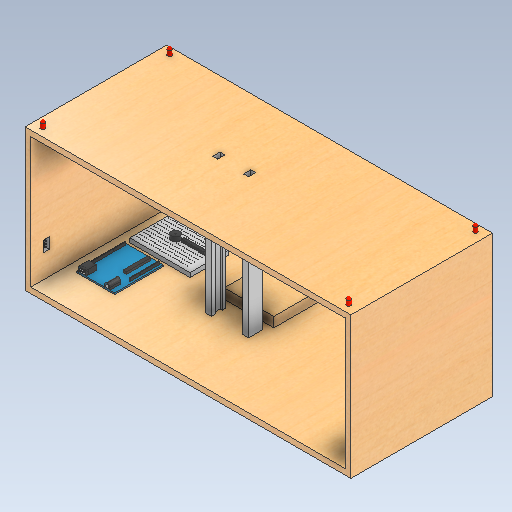
# Autodesk Inventor part: basement
Saved by Autodesk Inventor 2021 (Build 250183000, 183)
## iProperties
Created: 2021-06-27
Part Number: basement
Material: Generic
Document SubType Name: Modeling
Designer: TARUN
Density: 1 g/cm^3
Appearance: Default
Author: TARUN
Autodesk Inventor part; units mm, degrees
ref_plane "YZ Plane" through (0, 0, 0) normal (1, 0, 0) x (0, 1, 0)
ref_plane "XZ Plane" through (0, 0, 0) normal (0, 1, 0) x (-1, 0, 0)
ref_plane "XY Plane" through (0, 0, 0) normal (0, 0, 1) x (1, 0, 0)
sketch "Sketch1" plane through (0, 0, 0) normal (0, 0, 1) x (1, 0, 0)
  line L0 (-230, -100) -> (230, -100)
  line L1 (230, -100) -> (230, 100)
  line L2 (230, 100) -> (-230, 100)
  line L3 (-230, 100) -> (-230, -100)
  line L4 (-230, -100) -> (230, 100) construction
  line L5 (230, -100) -> (-230, 100) construction
  line L6 (222, 92) -> (222, -92)
  line L7 (222, -92) -> (-222, -92)
  line L8 (-222, -92) -> (-222, 92)
  line L9 (-222, 92) -> (222, 92)
  point P0 (0, 0)
  dimension "d0" = 460
  dimension "d1" = 200
  dimension "d2" = 8
  constraints: 20 end point, 4 parallel, 2 midpoint, 2 perpendicular, 1 horizontal, 3 other
  measures "d0" distance of L2.end L1.end
  measures "d1" distance of L1.end L0.end
  measures "d2" distance between parallel lines of L1 L6
extrude "Extrusion1" add sketch "Sketch1" along normal blind 200
sketch "Sketch2" plane through (-222, -92, 0) normal (0, 1, 0) x (1, 0, 0)
  line L0 (151.5163, -3.32) -> (221.5163, -3.32)
  line L1 (221.5163, -3.32) -> (221.5163, -78.32)
  line L2 (221.5163, -78.32) -> (151.5163, -78.32)
  line L3 (151.5163, -78.32) -> (151.5163, -3.32)
  line L4 (151.5163, -3.32) -> (221.5163, -78.32) construction
  line L5 (221.5163, -3.32) -> (151.5163, -78.32) construction
  line L6 (452, 0) -> (452, -200) projected
  line L7 (452, 0) -> (-8, 0) projected
  point P0 (222, 0)
  point P1 (186.5163, -40.82)
  dimension "d5" = 70
  dimension "d6" = 75
  constraints: 12 end point, 2 midpoint, 2 parallel, 1 horizontal, 1 perpendicular
  measures "d5" distance of L1.end L2.end
  measures "d6" distance of L0.end L1.end
extrude "Extrusion2" add sketch "Sketch2" along normal blind 14
sketch "Sketch4" plane through (-230, 100, 0) normal (0, 1, 0) x (1, 0, 0)
  line L0 (211.86, -103.32) -> (218.86, -103.32)
  line L1 (218.86, -103.32) -> (218.86, -93.32)
  line L2 (218.86, -93.32) -> (211.86, -93.32)
  line L3 (211.86, -93.32) -> (211.86, -103.32)
  line L4 (460, 0) -> (460, -200) projected
  line L5 (460, 0) -> (0, 0) projected
  line L6 (168.51, -103.32) -> (175.51, -103.32)
  line L7 (175.51, -103.32) -> (175.51, -93.32)
  line L8 (175.51, -93.32) -> (168.51, -93.32)
  line L9 (168.51, -93.32) -> (168.51, -103.32)
  point P0 (230, 0)
  dimension "d16" = 7
  dimension "d17" = 10
  dimension "d18" = 241.14
  dimension "d19" = 93.32
  dimension "d20" = 7
  dimension "d21" = 10
  dimension "d22" = 93.32
  dimension "d23" = 36.35
  constraints: 16 end point, 4 parallel, 2 horizontal, 2 perpendicular
  measures "d16" distance of L2.end L1.end
  measures "d17" distance of L1.end L0.end
  measures "d18" distance between parallel lines of L4 L1
  measures "d19" distance between parallel lines of L5 L2
  measures "d20" distance of L9.start L8.start
  measures "d21" distance of L8.start L6.end
  measures "d22" distance between parallel lines of L5 L8
  measures "d23" distance between parallel lines of L7 L3
extrude "Extrusion4" cut sketch "Sketch4" against normal blind 100
sketch "Sketch5" plane through (-222, -92, 0) normal (0, 1, 0) x (1, 0, 0)
  line L0 (163.51, -103.32) -> (160.51, -103.32)
  line L1 (160.51, -103.32) -> (160.51, -93.32)
  line L2 (160.51, -93.32) -> (163.51, -93.32)
  line L3 (163.51, -88.32) -> (155.51, -88.32)
  line L4 (155.51, -88.32) -> (155.51, -108.32)
  line L5 (155.51, -108.32) -> (163.51, -108.32)
  line L6 (163.51, -88.32) -> (163.51, -93.32)
  line L7 (163.51, -103.32) -> (163.51, -108.32)
  line L8 (452, -200) -> (-8, -200) projected
  line L9 (-8, 0) -> (-8, -200) projected
  line L10 (207.86, -103.32) -> (210.86, -103.32)
  line L11 (210.86, -103.32) -> (210.86, -93.32)
  line L12 (221.5163, -78.32) -> (151.5163, -78.32) projected
  line L13 (210.86, -93.32) -> (207.86, -93.32)
  line L14 (207.86, -88.32) -> (215.86, -88.32)
  line L15 (215.86, -88.32) -> (215.86, -108.32)
  line L16 (215.86, -108.32) -> (207.86, -108.32)
  line L17 (207.86, -108.32) -> (207.86, -103.32)
  line L18 (207.86, -93.32) -> (207.86, -88.32)
  point P0 (222, 0)
  dimension "d26" = 3
  dimension "d27" = 10
  dimension "d28" = 3
  dimension "d29" = 5
  dimension "d30" = 96.68
  dimension "d31" = 168.51
  dimension "d34" = 3
  dimension "d35" = 10
  dimension "d36" = 5
  dimension "d37" = 50.35
  dimension "d38" = 96.68
  constraints: 32 end point, 5 perpendicular, 3 horizontal, 2 collinear, 2 vertical, 4 other
  measures "d26" distance of L0.start L0.end
  measures "d27" distance of L0.end L1.end
  measures "d28" distance of L1.end L2.end
  measures "d29" distance between parallel lines of L2 L3
  measures "d30" distance between parallel lines of L8 L0
  measures "d31" distance between parallel lines of L9 L1
  measures "d34" distance of L10.start L10.end
  measures "d35" distance of L10.end L11.end
  measures "d36" distance between parallel lines of L11 L15
  measures "d37" distance between parallel lines of L11 L1
  measures "d38" distance between parallel lines of L8 L10
extrude "Extrusion5" add sketch "Sketch5" along normal blind 190
sketch "Sketch6" plane through (-222, -92, 0) normal (0, 1, 0) x (1, 0, 0)
  line L0 (15, -81.4) -> (68.4, -81.4)
  line L1 (68.4, -81.4) -> (68.4, -150)
  line L2 (68.4, -150) -> (15, -150)
  line L3 (15, -150) -> (15, -81.4)
  line L4 (0, 0) -> (0, -200) projected
  line L5 (452, -200) -> (-8, -200) projected
  point P0 (222, 0)
  dimension "d39" = 53.4
  dimension "d40" = 68.6
  dimension "d41" = 15
  dimension "d42" = 50
  constraints: 8 end point, 2 parallel, 1 horizontal, 1 perpendicular
  measures "d39" distance of L1.end L2.end
  measures "d40" distance of L0.end L1.end
  measures "d41" distance between parallel lines of L3 L4
  measures "d42" distance between parallel lines of L5 L2
extrude "Extrusion6" add sketch "Sketch6" along normal blind 2
sketch "Sketch7" plane through (-222, -90, 0) normal (0, 1, 0) x (1, 0, 0)
  line L0 (16.5988, -83.9592) -> (17.5988, -83.9592)
  line L1 (17.5988, -83.9592) -> (17.5988, -100.5861)
  line L2 (17.5988, -100.5861) -> (16.5988, -100.5861)
  line L3 (16.5988, -100.5861) -> (16.5988, -83.9592)
  line L4 (16.5988, -101.2096) -> (17.5988, -101.2096)
  line L5 (17.5988, -101.2096) -> (17.5988, -131.5683)
  line L6 (17.5988, -131.5683) -> (16.5988, -131.5683)
  line L7 (16.5988, -131.5683) -> (16.5988, -101.2096)
  line L8 (65.2067, -83.9592) -> (64.2067, -83.9592)
  line L9 (64.2067, -83.9592) -> (64.2067, -110.2877)
  line L10 (64.2067, -110.2877) -> (65.2067, -110.2877)
  line L11 (65.2067, -110.2877) -> (65.2067, -83.9592)
  line L12 (64.2067, -112.2693) -> (65.2067, -112.2693)
  line L13 (65.2067, -112.2693) -> (65.2067, -125.0662)
  line L14 (65.2067, -125.0662) -> (64.2067, -125.0662)
  line L15 (64.2067, -125.0662) -> (64.2067, -112.2693)
  line L16 (15, -150) -> (68.4, -150) projected
  line L17 (17.5988, -150) -> (27.1, -150)
  line L18 (27.1, -150) -> (27.1, -135.5269)
  line L19 (27.1, -135.5269) -> (17.5988, -135.5269)
  line L20 (17.5988, -135.5269) -> (17.5988, -150)
  line L21 (56.5691, -150) -> (64.2067, -150)
  line L22 (64.2067, -150) -> (64.2067, -135.5269)
  line L23 (64.2067, -135.5269) -> (56.5691, -135.5269)
  line L24 (56.5691, -135.5269) -> (56.5691, -150)
  line L25 (48.2496, -87.1807) -> (54.7806, -87.1807)
  line L26 (54.7806, -87.1807) -> (54.7806, -125.0662)
  line L27 (54.7806, -125.0662) -> (48.2496, -125.0662)
  line L28 (48.2496, -125.0662) -> (48.2496, -87.1807)
  point P0 (222, 0)
  dimension "d45" = 1
  dimension "d46" = 1
  constraints: 56 end point, 14 parallel, 11 point on line, 7 horizontal, 7 perpendicular
  measures "d45" distance of L1.end L2.end
  measures "d46" distance of L10.end L9.end
extrude "Extrusion7" add sketch "Sketch7" along normal blind 4 contours L0 L1 L2 L3 | L4 L5 L6 L7 | L11 L10 L9 L8 | L12 L13 L14 L15
sketch "Sketch8" plane through (-222, -90, 0) normal (0, 1, 0) x (1, 0, 0)
  line L0 (15, -150) -> (68.4, -150) projected
  line L1 (17.273, -150) -> (27.8568, -150)
  line L2 (27.8568, -150) -> (27.8568, -135.3219)
  line L3 (27.8568, -135.3219) -> (17.273, -135.3219)
  line L4 (17.273, -135.3219) -> (17.273, -150)
  line L5 (53.9943, -150) -> (61.6711, -150)
  line L6 (61.6711, -150) -> (61.6711, -134.54)
  line L7 (61.6711, -134.54) -> (53.9943, -134.54)
  line L8 (53.9943, -134.54) -> (53.9943, -150)
  point P0 (222, 0)
  constraints: 16 end point, 4 parallel, 2 horizontal, 2 perpendicular, 2 point on line
extrude "Extrusion8" add sketch "Sketch8" along normal blind 7
fillet "Fillet1" radius 3.83 2 edges at (-168.0057, -83, 142.27) (-160.3289, -83, 142.27)
sketch "Sketch9" plane through (-222, -90, 0) normal (0, 1, 0) x (1, 0, 0)
  line L0 (49.2469, -84.5196) -> (54.0315, -84.5196)
  line L1 (54.0315, -84.5196) -> (54.0315, -118.9701)
  line L2 (54.0315, -118.9701) -> (49.2469, -118.9701)
  line L3 (49.2469, -118.9701) -> (49.2469, -84.5196)
  point P0 (222, 0)
  constraints: 8 end point, 2 parallel, 1 horizontal, 1 perpendicular
extrude "Extrusion9" add sketch "Sketch9" along normal blind 3
sketch "Sketch10" plane through (-207, -92, 150) normal (0, 0, 1) x (1, 0, 0)
  line L0 (3.461, 2.8247) -> (3.461, 6.4078)
  line L1 (3.461, 6.4078) -> (4.9769, 8.0615)
  line L2 (4.9769, 8.0615) -> (10.4893, 8.0615)
  line L3 (10.4893, 8.0615) -> (12.062, 6.6199)
  line L4 (12.062, 6.6199) -> (12.062, 2.8247)
  line L5 (12.062, 2.8247) -> (3.461, 2.8247)
  line L6 (9.6853, 5.9944) -> (5.8863, 5.9944)
  line L7 (5.8863, 5.9944) -> (5.5282, 5.6037)
  line L8 (5.5282, 5.6037) -> (5.5282, 4.8919)
  line L9 (5.5282, 4.8919) -> (9.9949, 4.8919)
  line L10 (9.9949, 4.8919) -> (9.9949, 5.7105)
  line L11 (9.9949, 5.7105) -> (9.6853, 5.9944)
  circle A0 centre (42.8747, 4.6163) radius 2.2869
  point P0 (207, 92)
  constraints: 24 end point, 6 perpendicular, 2 parallel, 1 centre point, 1 vertical, 5 other
extrude "Extrusion10" cut sketch "Sketch10" against normal blind 4
sketch "Sketch11" plane through (-230, -100, 0) normal (-1, 0, 0) x (0, 0, 1)
  line L0 (173.8995, 56.6145) -> (182.7705, 56.6145)
  line L1 (182.7705, 56.6145) -> (182.7705, 41.1717)
  line L2 (182.7705, 41.1717) -> (173.8995, 41.1717)
  line L3 (173.8995, 41.1717) -> (173.8995, 56.6145)
  point P0 (0, 100)
  constraints: 8 end point, 2 parallel, 1 horizontal, 1 perpendicular
extrude "Extrusion11" add sketch "Sketch11" along normal blind 4
sketch "Sketch12" plane through (-234, -100, 0) normal (-1, 0, 0) x (0, 0, 1)
  line L0 (177.1802, 53.8974) -> (180.1802, 53.8974)
  line L1 (180.1802, 53.8974) -> (180.1802, 45.8974)
  line L2 (180.1802, 45.8974) -> (177.1802, 45.8974)
  line L3 (177.1802, 45.8974) -> (177.1802, 53.8974)
  point P0 (0, 100)
  dimension "d62" = 8
  dimension "d63" = 3
  constraints: 8 end point, 2 parallel, 1 horizontal, 1 perpendicular
  measures "d62" distance of L0.end L1.end
  measures "d63" distance of L1.end L2.end
extrude "Extrusion12" cut sketch "Sketch12" against normal blind 3
sketch "Sketch13" plane through (-231, -100, 0) normal (-1, 0, 0) x (0, 0, 1)
  line L0 (177.1802, 45.8974) -> (177.1802, 53.8974) projected
  line L1 (180.1802, 53.8974) -> (180.1802, 45.8974) projected
  line L2 (177.1802, 53.8974) -> (180.1802, 53.8974)
  line L3 (180.1802, 53.8974) -> (180.1802, 50.3139)
  line L4 (180.1802, 50.3139) -> (177.1802, 50.3139)
  line L5 (177.1802, 50.3139) -> (177.1802, 53.8974)
  point P0 (0, 100)
  constraints: 8 end point, 2 parallel, 1 horizontal, 1 perpendicular, 1 point on line
extrude "Extrusion13" add sketch "Sketch13" along normal blind 7
sketch "Sketch14" plane through (-222, -92, 0) normal (0, 1, 0) x (1, 0, 0)
  line L0 (15.7283, -20.9196) -> (100.7283, -20.9196)
  line L1 (100.7283, -20.9196) -> (100.7283, -75.9196)
  line L2 (100.7283, -75.9196) -> (15.7283, -75.9196)
  line L3 (15.7283, -75.9196) -> (15.7283, -20.9196)
  point P0 (222, 0)
  dimension "d64" = 85
  dimension "d65" = 55
  constraints: 8 end point, 2 parallel, 1 horizontal, 1 perpendicular
  measures "d64" distance of L1.end L2.end
  measures "d65" distance of L0.end L1.end
extrude "Extrusion14" add sketch "Sketch14" along normal blind 6
sketch "Sketch15" plane through (-222, -86, 0) normal (0, 1, 0) x (1, 0, 0)
  point P0 (222, 0)
  point P1 (18.7541, -24.4172)
hole "Hole1" at (-203.2459, -86, 24.4172) direction (0, -1, 0) diameter 1 depth 3
pattern_linear "Rectangular Pattern1" count 25 spacing 3 along (1, 0, 0) of "Hole1"
pattern_linear "Rectangular Pattern2" count 10 spacing 5 along (0, 0, 1) of "Hole1", "Rectangular Pattern1"
sketch "Sketch16" plane through (-222, -86, 0) normal (0, 1, 0) x (1, 0, 0)
  circle A0 centre (66.7541, -44.4172) radius 0.5 projected
  circle A1 centre (72.7541, -44.4172) radius 0.5 projected
  circle A2 centre (48.5894, -44.3397) radius 6.0208
  point P0 (222, 0)
  point P1 (72.6919, -43.9211)
  point P2 (72.7749, -44.9167)
  constraints: 1 centre point
extrude "Extrusion15" add sketch "Sketch16" along normal blind 6 contours A2
sketch "Sketch17" plane through (-173.4106, -80, 44.3397) normal (0, 1, 0) x (1, 0, 0)
  arc A0 (6.0077, 0.3972) -> (3.647, 4.7906) centre (0, 0) ccw projected
  circle A1 centre (0, 0) radius 0.7459
  point P0 (173.4106, 44.3397)
  point P1 (-2.5005, 5.477)
  point P2 (2.5005, 5.477)
  constraints: 1 centre point, 1 coincident
extrude "Extrusion16" cut sketch "Sketch17" against normal blind 1
sketch "Sketch18" plane through (-222, -86, 0) normal (0, 1, 0) x (1, 0, 0)
  line L0 (56.4403, -39.9172) -> (88.4242, -39.9172)
  line L1 (88.4242, -39.9172) -> (88.4242, -43.9172)
  line L2 (88.4242, -43.9172) -> (56.4403, -43.9172)
  line L3 (56.4403, -43.9172) -> (56.4403, -39.9172)
  point P0 (222, 0)
  constraints: 8 end point, 2 parallel, 1 horizontal, 1 perpendicular
extrude "Extrusion17" add sketch "Sketch18" along normal blind 3
sketch "Sketch19" plane through (-164.2459, -86, 43.9172) normal (0, 0, 1) x (1, 0, 0)
  line L0 (2.5, 2.2172) -> (2.5, 0)
  line L1 (0, 0) -> (3, 0) projected
  line L2 (2.5, 0) -> (3.5, 0) projected
  line L3 (3.5, 0) -> (3.5, 2.2172)
  line L4 (3.5, 2.2172) -> (2.5, 2.2172)
  line L5 (2.5, 0) -> (3.5, 0)
  line L6 (6, 0) -> (3, 0) projected
  line L7 (5.5, 0) -> (6.5, 0)
  line L8 (5.5, 2.2172) -> (5.5, 0)
  line L9 (6.5, 2.2172) -> (5.5, 2.2172)
  line L10 (6.5, 0) -> (6.5, 2.2172)
  line L11 (8.5, 0) -> (9.5, 0)
  line L12 (8.5, 2.2172) -> (8.5, 0)
  line L13 (9.5, 2.2172) -> (8.5, 2.2172)
  line L14 (9.5, 0) -> (9.5, 2.2172)
  line L15 (11.5, 0) -> (12.5, 0)
  line L16 (11.5, 2.2172) -> (11.5, 0)
  line L17 (12.5, 2.2172) -> (11.5, 2.2172)
  line L18 (12.5, 0) -> (12.5, 2.2172)
  line L19 (14.5, 0) -> (15.5, 0)
  line L20 (14.5, 2.2172) -> (14.5, 0)
  line L21 (15.5, 2.2172) -> (14.5, 2.2172)
  line L22 (15.5, 0) -> (15.5, 2.2172)
  line L23 (17.5, 0) -> (18.5, 0)
  line L24 (17.5, 2.2172) -> (17.5, 0)
  line L25 (18.5, 2.2172) -> (17.5, 2.2172)
  line L26 (18.5, 0) -> (18.5, 2.2172)
  line L27 (20.5, 0) -> (21.5, 0)
  line L28 (20.5, 2.2172) -> (20.5, 0)
  line L29 (21.5, 2.2172) -> (20.5, 2.2172)
  line L30 (21.5, 0) -> (21.5, 2.2172)
  line L31 (23.5, 0) -> (24.5, 0)
  line L32 (23.5, 2.2172) -> (23.5, 0)
  line L33 (24.5, 2.2172) -> (23.5, 2.2172)
  line L34 (24.5, 0) -> (24.5, 2.2172)
  line L35 (26.5, 0) -> (27.5, 0)
  line L36 (26.5, 2.2172) -> (26.5, 0)
  line L37 (27.5, 2.2172) -> (26.5, 2.2172)
  line L38 (27.5, 0) -> (27.5, 2.2172)
  point P0 (164.2459, 86)
  point P1 (5.5, 0)
  point P2 (6, 0)
  dimension "d89" = 3
  constraints: 72 end point, 2 collinear, 2 vertical, 1 horizontal, 1 perpendicular, 1 point on line, 63 other
  measures "d89" distance of L0.end L7.start
extrude "Extrusion18" add sketch "Sketch19" along normal blind 0.7
sketch "Sketch21" plane through (-134.2459, -86, 39.9172) normal (0, 0, -1) x (-1, 0, 0)
  line L0 (26.5, 0) -> (26.5, 2.2172) projected
  line L1 (26.5, 2.2172) -> (26.5, 0)
  line L2 (27, 0) -> (24, 0) projected
  line L3 (26.5, 2.2172) -> (27.5, 2.2172)
  line L4 (27.5, 2.2172) -> (27.5, 0)
  line L5 (30, 0) -> (27, 0) projected
  line L6 (26.5, 0) -> (27.5, 0)
  line L7 (23.5, 2.2172) -> (23.5, 0)
  line L8 (23.5, 2.2172) -> (24.5, 2.2172)
  line L9 (24.5, 2.2172) -> (24.5, 0)
  line L10 (23.5, 0) -> (24.5, 0)
  line L11 (20.5, 2.2172) -> (20.5, 0)
  line L12 (20.5, 2.2172) -> (21.5, 2.2172)
  line L13 (21.5, 2.2172) -> (21.5, 0)
  line L14 (20.5, 0) -> (21.5, 0)
  line L15 (17.5, 2.2172) -> (17.5, 0)
  line L16 (17.5, 2.2172) -> (18.5, 2.2172)
  line L17 (18.5, 2.2172) -> (18.5, 0)
  line L18 (17.5, 0) -> (18.5, 0)
  line L19 (14.5, 2.2172) -> (14.5, 0)
  line L20 (14.5, 2.2172) -> (15.5, 2.2172)
  line L21 (15.5, 2.2172) -> (15.5, 0)
  line L22 (14.5, 0) -> (15.5, 0)
  line L23 (11.5, 2.2172) -> (11.5, 0)
  line L24 (11.5, 2.2172) -> (12.5, 2.2172)
  line L25 (12.5, 2.2172) -> (12.5, 0)
  line L26 (11.5, 0) -> (12.5, 0)
  line L27 (8.5, 2.2172) -> (8.5, 0)
  line L28 (8.5, 2.2172) -> (9.5, 2.2172)
  line L29 (9.5, 2.2172) -> (9.5, 0)
  line L30 (8.5, 0) -> (9.5, 0)
  line L31 (5.5, 2.2172) -> (5.5, 0)
  line L32 (5.5, 2.2172) -> (6.5, 2.2172)
  line L33 (6.5, 2.2172) -> (6.5, 0)
  line L34 (5.5, 0) -> (6.5, 0)
  line L35 (2.5, 2.2172) -> (2.5, 0)
  line L36 (2.5, 2.2172) -> (3.5, 2.2172)
  line L37 (3.5, 2.2172) -> (3.5, 0)
  line L38 (2.5, 0) -> (3.5, 0)
  point P0 (-134.2459, 86)
  point P1 (24, 0)
  point P2 (24.5, 0)
  dimension "d98" = 3
  constraints: 72 end point, 3 horizontal, 2 point on line, 1 collinear, 1 perpendicular, 1 vertical, 63 other
  measures "d98" distance of L0.end L7.start
extrude "Extrusion19" add sketch "Sketch21" along normal blind 0.7
sketch "Sketch22" plane through (-230, -100, 0) normal (-1, 0, 0) x (0, 0, 1)
  line L0 (182.7705, 56.6145) -> (182.7705, 41.1717) projected
  line L1 (173.8995, 56.6145) -> (182.7705, 56.6145)
  line L2 (182.7705, 56.6145) -> (182.7705, 41.1717)
  line L3 (182.7705, 41.1717) -> (173.8995, 41.1717)
  line L4 (173.8995, 41.1717) -> (173.8995, 56.6145)
  point P0 (0, 100)
  constraints: 8 end point, 2 parallel, 1 horizontal, 1 perpendicular
extrude "Extrusion20" cut sketch "Sketch22" against normal blind 10
sketch "Sketch23" plane through (-230, -100, 0) normal (1, 0, 0) x (0, 0, -1)
  line L0 (-177.5509, 52.7622) -> (-176.6229, 52.7622)
  line L1 (-176.6229, 52.7622) -> (-176.6229, 51.8319)
  line L2 (-176.6229, 51.8319) -> (-177.5509, 51.8319)
  line L3 (-177.5509, 51.8319) -> (-177.5509, 52.7622)
  line L4 (-177.5509, 48.7622) -> (-176.6229, 48.7622)
  line L5 (-176.6229, 48.7622) -> (-176.6229, 47.8319)
  line L6 (-177.5509, 47.8319) -> (-177.5509, 48.7622)
  line L7 (-176.6229, 47.8319) -> (-177.5509, 47.8319)
  line L8 (-177.5509, 44.7622) -> (-176.6229, 44.7622)
  line L9 (-176.6229, 44.7622) -> (-176.6229, 43.8319)
  line L10 (-177.5509, 43.8319) -> (-177.5509, 44.7622)
  line L11 (-176.6229, 43.8319) -> (-177.5509, 43.8319)
  point P0 (0, 100)
  dimension "d109" = 4
  constraints: 24 end point, 2 parallel, 1 collinear, 1 horizontal, 1 perpendicular, 1 vertical, 15 other
  measures "d109" distance of L0.start L4.start
extrude "Extrusion21" add sketch "Sketch23" along normal blind 7
sketch "Sketch24" plane through (-230, 100, 0) normal (0, 1, 0) x (1, 0, 0)
  circle A0 centre (14, -10) radius 3
  line L0 (0, 0) -> (0, -200) projected
  line L1 (460, 0) -> (0, 0) projected
  circle A1 centre (446, -10) radius 3
  circle A2 centre (14, -189) radius 3
  circle A3 centre (446, -189) radius 3
  point P0 (230, 0)
  dimension "d116" = 6
  dimension "d120" = 14
  dimension "d121" = 10
  dimension "d124" = 432
  dimension "d131" = 179
  constraints: 4 centre point, 1 horizontal, 1 vertical, 6 other
  measures "d116" diameter of A0
  measures "d120" distance from line of L0 A0.centre
  measures "d121" distance from line of A0.centre L1
  measures "d124" distance of A0.centre A1.centre
  measures "d131" distance of A0.centre A2.centre
extrude "Extrusion22" add sketch "Sketch24" along normal blind 10
fillet "Fillet2" radius 3 4 edges at (-219, 110, 10) (213, 110, 189) (213, 110, 10) (-219, 110, 189)
body "Solid1"
